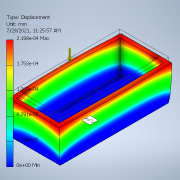
# Autodesk Inventor part: Stress analysis
Saved by Autodesk Inventor 2021 (Build 250183000, 183)
## iProperties
Created: 2021-07-29
Part Number: Stress analysis
Material: Aluminum 6061-AHC
Document SubType Name: Modeling
Designer: Shammy Haider
Density: 2.7 g/cm^3
Sheet Metal Width: 0.000 mm
Sheet Metal Length: 0.000 mm
Sheet Metal Area: 0.000 mm^2
Appearance: Aluminum - Dark
Author: Shammy Haider
Autodesk Inventor part; units mm, degrees
ref_plane "YZ Plane" through (0, 0, 0) normal (1, 0, 0) x (0, 1, 0)
ref_plane "XZ Plane" through (0, 0, 0) normal (0, 1, 0) x (-1, 0, 0)
ref_plane "XY Plane" through (0, 0, 0) normal (0, 0, 1) x (1, 0, 0)
sketch "Sketch1" plane through (0, 0, 0) normal (0, 1, 0) x (-1, 0, 0)
  line L0 (6.0929, 13.5835) -> (-6.0929, 13.5835)
  line L1 (-6.0929, 13.5835) -> (-6.0929, -13.5835)
  line L2 (-6.0929, -13.5835) -> (6.0929, -13.5835)
  line L3 (6.0929, -13.5835) -> (6.0929, 13.5835)
  line L4 (6.0929, 13.5835) -> (-6.0929, -13.5835) construction
  line L5 (-6.0929, 13.5835) -> (6.0929, -13.5835) construction
  point P0 (0, 0)
  constraints: 12 end point, 2 midpoint, 2 parallel, 1 horizontal, 1 perpendicular
extrude "Extrusion1" add sketch "Sketch1" along normal blind 10
shell "Shell1" thickness 1 removed faces 1 at (2.031, 10, -4.5278)
equation "\"BendRadius\" = Thickness"
equation "\"BendReliefWidth\" = Thickness"
equation "\"BendReliefDepth\" = 0.5 * Thickness"
equation "\"CornerReliefSize\" = 4 * Thickness"
equation "\"MinimumRemnant\" = 2 * Thickness"
equation "\"TransitionRadius\" = BendRadius"
equation "\"JacobiRadiusSize\" = BendRadius"
equation "\"GapSize\" = Thickness"
equation "\"Thickness\" = 1"
body "Solid1"
